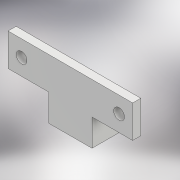
# Autodesk Inventor part: DefaultMotorMountBack
Saved by Autodesk Inventor 2018.2 (Build 222227000, 227)
## iProperties
Created: 2018-03-31
Part Number: DefaultMotorMountBack
Material: ABS Plastic
Document SubType Name: Modeling
Designer: Muchen He
Density: 1.06 g/cm^3
Appearance: Smooth - White
Author: Muchen He
Autodesk Inventor part; units mm, degrees
ref_plane "YZ Plane" through (0, 0, 0) normal (1, 0, 0) x (0, 1, 0)
ref_plane "XZ Plane" through (0, 0, 0) normal (0, 1, 0) x (-1, 0, 0)
ref_plane "XY Plane" through (0, 0, 0) normal (0, 0, 1) x (1, 0, 0)
sketch "Sketch1" plane through (0, 0, 0) normal (0, 0, 1) x (1, 0, 0)
  arc A0 (0, 12) -> (8, 14.5109) centre (0, 26) ccw
  line L0 (0, 0) -> (0, 12) construction
  line L1 (8, 14.5109) -> (8, 0)
  arc A1 (-8, 14.5109) -> (0, 12) centre (0, 26) ccw
  line L2 (-8, 14.5109) -> (-8, 0)
  line L3 (-8, 0) -> (0, 0)
  line L4 (0, 0) -> (8, 0)
  dimension "d0" = 14
  dimension "d9" = 8
  dimension "d13" = 26
  constraints: 10 end point, 4 point on circle, 2 centre point, 2 horizontal, 2 symmetric about line, 2 vertical, 2 vertical alignment, 1 coincident, 1 other
  measures "d0" radius of A0
  measures "d9" distance between parallel lines of L0 L1
  measures "d13" distance from line of L3 A0.centre
extrude "Extrusion1" add sketch "Sketch1" along normal blind 10
sketch "Sketch2" plane through (-8, 0, 0) normal (0, -1, 0) x (1, 0, 0)
  circle A0 centre (-10, 16) radius 2
  circle A1 centre (26, 16) radius 2
  line L0 (-10, 16) -> (26, 16) construction
  line L1 (16, 0) -> (0, 0) construction
  line L2 (0, 10) -> (16, 10) construction
  line L3 (-15, 22) -> (31, 22)
  line L4 (31, 22) -> (31, 10)
  line L5 (31, 10) -> (-15, 10)
  line L6 (-15, 10) -> (-15, 22)
  point P0 (8, 0)
  point P1 (8, 16)
  point P2 (8, 0)
  point P3 (31, 16)
  point P4 (8, 22)
  dimension "d14" = 4
  dimension "d15" = 4
  dimension "d16" = 36
  dimension "d17" = 6
  dimension "d18" = 46
  constraints: 10 end point, 4 midpoint, 2 centre point, 2 horizontal, 2 horizontal alignment, 2 parallel, 2 vertical alignment, 1 perpendicular
  measures "d14" diameter of A1
  measures "d15" diameter of A0
  measures "d16" distance of L0.start L0.end
  measures "d17" distance between parallel lines of L2 L0
  measures "d18" distance of L3.start L3.end
extrude "Extrusion2" add sketch "Sketch2" against normal blind 3
body "Solid1"
